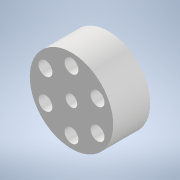
# Autodesk Inventor part: servo shaft flange
Saved by Autodesk Inventor 2021 (Build 250183000, 183)
## iProperties
Created: 2021-11-23
Part Number: servo shaft flange
Material: Generic
Document SubType Name: Modeling
Designer: techv
Density: 1 g/cm^3
Appearance: Default
Author: techv
Autodesk Inventor part; units mm, degrees
ref_plane "YZ Plane" through (0, 0, 0) normal (1, 0, 0) x (0, 1, 0)
ref_plane "XZ Plane" through (0, 0, 0) normal (0, 1, 0) x (-1, 0, 0)
ref_plane "XY Plane" through (0, 0, 0) normal (0, 0, 1) x (1, 0, 0)
sketch "Sketch1" plane through (0, 0, 0) normal (0, 0, 1) x (1, 0, 0)
  circle A0 centre (0, 0) radius 4 projected
  circle A1 centre (0, 0) radius 9
  point P0 (0, 0)
  dimension "d0" = 18
  constraints: 1 centre point, 1 coincident
  measures "d0" diameter of A1
extrude "Extrusion1" add sketch "Sketch1" along normal blind 3 and the other way blind 5 contours A0 | A1
sketch "Sketch2" plane through (0, 0, 3) normal (0, 0, 1) x (1, 0, 0)
  circle A0 centre (0, 0) radius 6.5 construction
  circle A1 centre (0, 6.5) radius 1.5
  circle A2 centre (-5.6292, 3.25) radius 1.5
  circle A3 centre (-5.6292, -3.25) radius 1.5
  circle A4 centre (0, -6.5) radius 1.5
  circle A5 centre (5.6292, -3.25) radius 1.5
  circle A6 centre (5.6292, 3.25) radius 1.5
  dimension "d5" = 13
  dimension "d6" = 3
  dimension "d9" = 360
  constraints: 6 centre point, 1 coincident, 1 vertical alignment, 15 other
  measures "d6" diameter of A1
extrude "Extrusion2" cut sketch "Sketch2" against normal through all
sketch "Sketch3" plane through (0, 0, 3) normal (0, 0, 1) x (1, 0, 0)
  circle A0 centre (0, 0) radius 1.25
  dimension "d13" = 2.5
  constraints: 1 centre point, 1 coincident
  measures "d13" diameter of A0
extrude "Extrusion3" cut sketch "Sketch3" against normal through all
body "Solid1"
